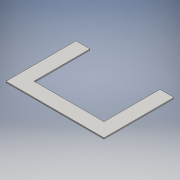
# Autodesk Inventor part: OuterFrame
Saved by Autodesk Inventor 2016 (Build 200138000, 138)
## iProperties
Created: 2016-05-22
Part Number: OuterFrame
Material: Generic
Document SubType Name: Modeling
Designer: Kurtis
Density: 1 g/cm^3
Appearance: Default
Author: Kurtis
Autodesk Inventor part; units mm, degrees
ref_plane "YZ Plane" through (0, 0, 0) normal (1, 0, 0) x (0, 1, 0)
ref_plane "XZ Plane" through (0, 0, 0) normal (0, 1, 0) x (-1, 0, 0)
ref_plane "XY Plane" through (0, 0, 0) normal (0, 0, 1) x (1, 0, 0)
sketch "Sketch1" plane through (0, 0, 0) normal (0, 0, 1) x (1, 0, 0)
  line L0 (0, 0) -> (420, 0)
  line L1 (420, 0) -> (420, 300)
  line L2 (420, 300) -> (360, 300)
  line L3 (360, 300) -> (360, 60)
  line L4 (360, 60) -> (60, 60)
  line L5 (60, 60) -> (60, 300)
  line L6 (60, 300) -> (0, 300)
  line L7 (0, 300) -> (0, 0)
  line L8 (0, 300) -> (0, 240) construction
  line L9 (0, 240) -> (0, 180) construction
  line L10 (0, 180) -> (0, 120) construction
  line L11 (0, 120) -> (0, 60) construction
  line L12 (420, 300) -> (420, 240) construction
  line L13 (420, 240) -> (420, 180) construction
  line L14 (420, 180) -> (420, 120) construction
  line L15 (420, 120) -> (420, 60) construction
  line L16 (60, 60) -> (120, 60) construction
  line L17 (120, 60) -> (180, 60) construction
  line L18 (180, 60) -> (240, 60) construction
  line L19 (240, 60) -> (300, 60) construction
  line L20 (300, 60) -> (360, 60) construction
  line L21 (0, 240) -> (60, 300) construction
  line L22 (0, 240) -> (60, 240) construction
  line L23 (0, 180) -> (60, 180) construction
  line L24 (0, 120) -> (60, 120) construction
  line L25 (0, 60) -> (60, 60) construction
  line L26 (60, 60) -> (60, 0) construction
  line L27 (0, 180) -> (60, 240) construction
  line L28 (0, 120) -> (60, 180) construction
  line L29 (0, 60) -> (60, 120) construction
  line L30 (0, 0) -> (60, 60) construction
  line L31 (120, 60) -> (120, 0) construction
  line L32 (180, 60) -> (180, 0) construction
  line L33 (240, 60) -> (240, 0) construction
  line L34 (300, 60) -> (300, 0) construction
  line L35 (360, 60) -> (360, 0) construction
  line L36 (360, 60) -> (420, 60) construction
  line L37 (360, 120) -> (420, 120) construction
  line L38 (420, 180) -> (360, 180) construction
  line L39 (420, 240) -> (360, 240) construction
  line L40 (60, 0) -> (120, 60) construction
  line L41 (120, 0) -> (180, 60) construction
  line L42 (180, 0) -> (240, 60) construction
  line L43 (240, 0) -> (300, 60) construction
  line L44 (300, 0) -> (360, 60) construction
  line L45 (360, 0) -> (420, 60) construction
  line L46 (360, 60) -> (420, 120) construction
  line L47 (360, 120) -> (420, 180) construction
  line L48 (360, 180) -> (420, 240) construction
  line L49 (360, 240) -> (420, 300) construction
  dimension "d0" = 420
  dimension "d1" = 300
  dimension "d2" = 60
  dimension "d3" = 240
  dimension "d4" = 300
  dimension "d5" = 240
  dimension "d6" = 60
  dimension "d7" = 60
  dimension "d8" = 60
  dimension "d9" = 60
  dimension "d10" = 60
  dimension "d11" = 60
  dimension "d12" = 60
  dimension "d13" = 60
  dimension "d14" = 60
  dimension "d15" = 60
  dimension "d16" = 60
  dimension "d17" = 60
  constraints: 100 end point, 29 point on line, 14 perpendicular, 2 equal length, 2 horizontal, 2 midpoint
  measures "d0" distance of L0.start L0.end
  measures "d1" distance of L0.end L1.end
  measures "d2" distance of L1.end L2.end
  measures "d3" distance of L2.end L3.end
  measures "d4" distance of L3.end L4.end
  measures "d5" distance of L4.end L5.end
  measures "d6" distance of L6.end L8.end
  measures "d7" distance of L8.end L9.end
  measures "d8" distance of L9.end L10.end
  measures "d9" distance of L10.end L11.end
  measures "d10" distance of L1.end L12.end
  measures "d11" distance of L12.end L13.end
  measures "d12" distance of L13.end L14.end
  measures "d13" distance of L14.end L15.end
  measures "d14" distance of L4.end L16.end
  measures "d15" distance of L16.end L17.end
  measures "d16" distance of L17.end L18.end
  measures "d17" distance of L18.end L19.end
extrude "Extrusion1" add sketch "Sketch1" along normal blind 5
body "Solid1"
